TS100 Soldering Iron Clip (Autodesk Fusion 360 design; units mm, degrees)
Autodesk Fusion 360 part; units mm, degrees
note: some values were not read from the file. Chosen so that the rebuilt part matches the saved one: which pieces of a blend or face edit are solid.
sketch "Sketch Silhouette of tool" plane through (0, 0, 0) normal (0, 0, 1) x (1, 0, 0)
  line L0 (0, 0) -> (0, 9.5) construction
  line L1 (3.2731, 9.5) -> (6.0561, 2.3608)
  line L2 (-3.2731, 9.5) -> (-6.0561, 2.3608)
  line L3 (3.2731, 9.5) -> (-3.2731, 9.5)
  arc A0 (-6.0561, 2.3608) -> (6.0561, 2.3608) centre (0, 0) ccw
  dimension "d1" = 13
  dimension "d2" = 9.5
  dimension "d3" = 6.5462
  constraint coincident L0.start A0.centre
  constraint tangent L1 A0
  constraint symmetric L0 L1.start L2.start
  constraint symmetric L0 L1.end L2.end
  constraint coincident L0.end L3
  constraint horizontal L3
  measures "d1" diameter of A0
  measures "d2" distance of L0.start L0.end
  measures "d3" distance of L1.start L2.start
sketch "Sketch Tool Holder" plane through (0, 0, 0) normal (0, 0, 1) x (1, 0, 0)
  arc A0 (-6.0561, 2.3608) -> (6.0561, 2.3608) centre (0, 0) ccw
  arc A1 (0, -7) -> (7, 0) centre (0, 0) ccw
  line L0 (7, 0) -> (4.1528, 6.3948)
  line L1 (4.1528, 6.3948) -> (4.7008, 7.5183)
  line L2 (5.5996, 7.0799) -> (5.2561, 6.3756)
  line L3 (4.7008, 7.5183) -> (5.5996, 7.0799) construction
  line L4 (5.2561, 6.3756) -> (9.8756, -4)
  line L5 (0, 0) -> (0, -10.7856) construction
  line L6 (0, 0) -> (7, 0)
  line L7 (7, 0) -> (7, -1.099) construction
  arc A2 (5.5996, 7.0799) -> (4.7008, 7.5183) centre (5.1502, 7.2991) ccw
  line L8 (0, -10) -> (9.8756, -10)
  line L9 (9.8756, -10) -> (9.8756, -4)
  line L10 (-7, 0) -> (-4.1528, 6.3948)
  line L11 (-4.1528, 6.3948) -> (-4.7008, 7.5183)
  arc A3 (-4.7008, 7.5183) -> (-5.5996, 7.0799) centre (-5.1502, 7.2991) ccw
  line L12 (-5.5996, 7.0799) -> (-5.2561, 6.3756)
  line L13 (-5.2561, 6.3756) -> (-9.8756, -4)
  line L14 (-9.8756, -10) -> (-9.8756, -4)
  line L15 (0, -10) -> (-9.8756, -10)
  arc A4 (-7, 0) -> (0, -7) centre (0, 0) ccw
  dimension "d7" = 0.5
  dimension "d8" = 1
  dimension "d9" = 1
  dimension "d10" = 130
  dimension "d11" = 66
  dimension "d12" = 1.25
  dimension "d14" = 7
  dimension "d15" = 3
  dimension "d16" = 6
  constraint parallel L1 L2
  constraint perpendicular L1 L3
  constraint concentric A0 A1
  constraint parallel L0 L4
  constraint coincident A0.centre A1.centre
  constraint vertical L5
  constraint coincident A1 L0.start
  constraint perpendicular L5 L6
  constraint tangent A1 L7
  constraint tangent L1 A2
  constraint coincident L5 L8.start
  constraint perpendicular L5 L8
  constraint perpendicular L8 L9
  constraint symmetric A1.start L5 A4.end
  constraint symmetric A1 L5 A4
  constraint symmetric L0.end L5 L10.end
  constraint symmetric L1.end L5 L11.end
  constraint symmetric L2.start L5 A3.end
  constraint symmetric L2.end L5 L12.end
  constraint symmetric L4.end L5 L13.end
  constraint symmetric L5 A1.end L10.start
  constraint symmetric L5 A2 A3
  constraint symmetric L5 L8.start L15.start
  constraint symmetric L5 L8.end L14.start
  measures "d7" distance of A0 A1
  measures "d8" distance of L0 L4
  measures "d9" distance of L1 L2
  measures "d10" angle of L0 L1
  measures "d11" angle of L0 L6
  measures "d12" distance of L0.end L1.end
  measures "d14" distance of L0.end A1.end
  measures "d15" distance of L8.start A1.start
  measures "d16" distance of L4.end L8.end
extrude "Extrude1" add sketch "Sketch Tool Holder" along normal blind 13 contours A1 L0 L1 L2 L4 A2 L8 L9 L10 L11 A3 L12 L13 L14 L15 A4
fillet "Fillet1" radius 4 8 edges at (-7, 0, 6.5) (7, 0, 6.5) (-9.8756, -4, 6.5) (9.8756, -4, 6.5) (4.1528, 6.3948, 6.5) (-4.1528, 6.3948, 6.5) (5.2561, 6.3756, 6.5) (-5.2561, 6.3756, 6.5)
equation "d2 = 16 mm - ( 0.5 * d1 )"
named bodies: "Ts100 soldering iron clip"
